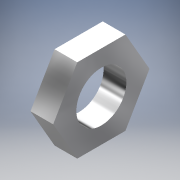
# Autodesk Inventor part: Stopper Outer
Saved by Autodesk Inventor 2019.4 (Build 234330000, 330)
## iProperties
Created: 2020-03-11
Part Number: Stopper Outer
Material: Aluminum 6061
Document SubType Name: Modeling
Designer: Mark
Mass: 43.3087 g
Surface Area: 58.5839 cm^2
Volume: 16.0403 cm^3
Density: 2.7 g/cm^3
Appearance: Aluminum - Flat
Author: Mark
Autodesk Inventor part; units mm, degrees
ref_plane "YZ Plane" through (0, 0, 0) normal (1, 0, 0) x (0, 1, 0)
ref_plane "XZ Plane" through (0, 0, 0) normal (0, 1, 0) x (-1, 0, 0)
ref_plane "XY Plane" through (0, 0, 0) normal (0, 0, 1) x (1, 0, 0)
sketch "Sketch1" plane through (0, 0, 0) normal (1, 0, 0) x (0, 1, 0)
  circle A0 centre (0, 0) radius 15
  line L0 (25, -14.4338) -> (0, -28.8675)
  line L1 (0, -28.8675) -> (-25, -14.4338)
  line L2 (-25, -14.4338) -> (-25, 14.4338)
  line L3 (-25, 14.4338) -> (0, 28.8675)
  line L4 (0, 28.8675) -> (25, 14.4338)
  line L5 (25, 14.4338) -> (25, -14.4338)
  line L6 (0, 0) -> (25, 0)
  line L7 (0, 0) -> (25, 0) construction
  dimension "d0" = 30
  dimension "d1" = 25
  dimension "d2" = 25
  dimension "d3" = 0
  dimension "d4" = 90
  constraints: 16 end point, 2 coincident, 2 horizontal, 1 centre point, 1 collinear, 13 other
  measures "d0" diameter of A0
  measures "d1" distance from line of point (0, 0) L5
  measures "d2" distance of L6.start L6.end
  measures "d3" distance between parallel lines of L6 L7
  measures "d4" angle of L5 L6
extrude "Extrusion1" add sketch "Sketch1" along normal blind 13.6
body "Solid1"
